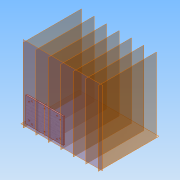
# Autodesk Inventor part: Selection_Ramp 1 2 Lanes
Saved by Autodesk Inventor 2018.1 (Build 221171000, 171)
## iProperties
Created: 2019-02-07
Part Number: Selection_Ramp 1 2 Lanes
Material: Wood (Oak)
Document SubType Name: Modeling
Designer: James
Density: 0.76 g/cm^3
Appearance: White Oak - Natural Medium Gloss
Author: James
Autodesk Inventor part; units mm, degrees
ref_plane "YZ Plane" through (0, 0, 0) normal (1, 0, 0) x (0, 1, 0)
ref_plane "XZ Plane" through (0, 0, 0) normal (0, 1, 0) x (-1, 0, 0)
ref_plane "XY Plane" through (0, 0, 0) normal (0, 0, 1) x (1, 0, 0)
derived "Selection_Skeleton.ipt"
ref_plane "Ground" through (0, 0, 0) normal (0, 1, 0) x (-1, 0, 0)
ref_plane "LHS inner" through (0, 0, 0) normal (1, 0, 0) x (0, 1, 0)
ref_plane "RHS inner" through (300, 0, 0) normal (1, 0, 0) x (0, 1, 0)
ref_plane "Lane 1" through (50, 0, 0) normal (1, 0, 0) x (0, 1, 0)
ref_plane "Lane 2" through (100, 0, 0) normal (1, 0, 0) x (0, 1, 0)
ref_plane "Lane 3" through (150, 0, 0) normal (1, 0, 0) x (0, 1, 0)
ref_plane "Lane 4" through (200, 0, 0) normal (1, 0, 0) x (0, 1, 0)
ref_plane "Lane 5" through (250, 0, 0) normal (1, 0, 0) x (0, 1, 0)
ref_plane "Back" through (0, 0, 0) normal (0, 0, 1) x (1, 0, 0)
sketch "Sketch1" plane through (0, 0, 0) normal (0, 1, 0) x (-1, 0, 0)
  line L0 (0, -20) -> (0, 120) projected
  line L1 (-180, 0) -> (30, 0) projected
  line L2 (0, 0) -> (-150, 0)
  line L3 (-150, 0) -> (-150, 100)
  line L4 (-150, 100) -> (0, 100)
  line L5 (0, 100) -> (0, 0)
  line L6 (-150, -20) -> (-150, 120) projected
  dimension "d1" = 100
  constraints: 8 end point, 2 parallel, 1 collinear, 1 horizontal, 1 perpendicular
  measures "d1" distance of L2.end L3.end
extrude "Extrusion1" add sketch "Sketch1" along normal blind 5
sketch "Sketch2" plane through (0, 5, 0) normal (0, 1, 0) x (1, 0, 0)
  line L0 (150, 0) -> (0, 0) projected
  line L1 (0, -100) -> (150, -100) projected
  line L2 (50, 20) -> (50, -120) projected
  point P0 (25, -10)
  point P1 (25, -90)
  dimension "d4" = 10
  dimension "d5" = 10
  dimension "d6" = 80
  dimension "d7" = 25
  constraints: 1 vertical alignment
  measures "d4" distance from line of point (25, -10) L0
  measures "d5" distance from line of L1 point (25, -90)
  measures "d6" distance of point (25, -10) point (25, -90)
  measures "d7" distance from line of L2 point (25, -10)
hole "Hole1" at (25, 5, 10) at (25, 5, 90) direction (0, -1, 0) diameter 4.5 end through all clearance for "Socket Head Cap Screw" size "M4" standard "Ansi Metric M Profile"
pattern_linear "Rectangular Pattern1" count 3 spacing 50 along (1, 0, 0) of "Hole1"
ref_plane "Mid Plane" through (75, 0, 0) normal (-1, 0, 0) x (0, 0, 1)
sketch "Sketch4" plane through (0, 5, 0) normal (0, 1, 0) x (1, 0, 0)
  line L0 (0, 0) -> (0, -100) projected
  line L1 (150, 0) -> (0, 0) projected
  line L2 (0, -100) -> (150, -100) projected
  point P0 (12.5, -17.5)
  point P1 (12.5, -82.5)
  dimension "d29" = 12.5
  dimension "d30" = 65
  dimension "d31" = 17.5
  dimension "d32" = 17.5
  constraints: 1 vertical alignment
  measures "d29" distance from line of L0 point (12.5, -17.5)
  measures "d30" distance of point (12.5, -17.5) point (12.5, -82.5)
  measures "d31" distance from line of L1 point (12.5, -17.5)
  measures "d32" distance from line of L2 point (12.5, -82.5)
hole "Hole3" at (12.5, 5, 17.5) at (12.5, 5, 82.5) direction (0, -1, 0) diameter 4.5 end through all countersink diameter 9.4 countersink angle 90 clearance for "Flat Head Machine Screw" size "M4" standard "Ansi Metric M Profile"
mirror "Mirror2" about plane through (75, 0, 0) normal (-1, 0, 0) of "Hole3"
equation "\"d5\" = d4"
equation "\"d31\" = d32"
body "Solid1"
